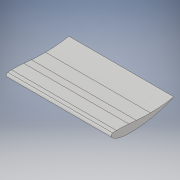
# Autodesk Inventor part: naca97
Saved by Autodesk Inventor 2018.2 (Build 222227000, 227)
## iProperties
Created: 2018-02-23
Part Number: naca97
Material: 一般
Document SubType Name: Modeling
Designer: ku_sk
Density: 1 g/cm^3
Appearance: 既定
Author: ku_sk
Autodesk Inventor part; units mm, degrees
ref_plane "YZ Plane" through (0, 0, 0) normal (1, 0, 0) x (0, 1, 0)
ref_plane "XZ Plane" through (0, 0, 0) normal (0, 1, 0) x (-1, 0, 0)
ref_plane "XY Plane" through (0, 0, 0) normal (0, 0, 1) x (1, 0, 0)
sketch "スケッチ1" plane through (0, 0, 0) normal (0, 1, 0) x (-1, 0, 0)
  arc A0 (-0.3139, 1.7491) -> (-1.4341, -1.0494) centre (0, 0) ccw
  arc A1 (3.0473, 2.0538) -> (-0.3139, 1.7491) centre (3.11, -17.328) ccw
  arc A2 (14.2243, 1.5555) -> (3.0473, 2.0538) centre (3.426, -115.066) ccw
  arc A3 (14.2243, 1.5555) -> (21.0741, 0.9324) centre (210.779, 2124.35) ccw
  arc A4 (21.0741, 0.9324) -> (33.8498, 0.3962) centre (33.144, 136.034) ccw
  arc A5 (33.8498, 0.3962) -> (55, 2.3978) centre (33.229, 119.698) ccw
  arc A6 (-1.4341, -1.0494) -> (-0.1426, -2.3034) centre (2.9, 2.122) ccw
  arc A7 (-0.1426, -2.3034) -> (4.4066, -4.5379) centre (9.743, 12.075) ccw
  arc A8 (4.4066, -4.5379) -> (12.2873, -5.9387) centre (13.508, 23.796) ccw
  arc A9 (12.2873, -5.9387) -> (16.5781, -5.9878) centre (15.261, 66.497) ccw
  arc A10 (16.5781, -5.9878) -> (55, 2.3978) centre (14.7503, 94.6026) ccw
  dimension "d0" = 1.777
  dimension "d2" = 17.328
  dimension "d5" = 115.066
  dimension "d7" = 2124.35
  dimension "d9" = 136.034
  dimension "d10" = 3.11
  dimension "d11" = 3.426
  dimension "d12" = 210.779
  dimension "d13" = 33.144
  dimension "d14" = 33.229
  dimension "d15" = 119.698
  dimension "d16" = 55
  dimension "d17" = 2.9
  dimension "d18" = 2.122
  dimension "d21" = 9.743
  dimension "d22" = 12.075
  dimension "d23" = 13.508
  dimension "d24" = 23.796
  dimension "d25" = 15.261
  dimension "d26" = 66.497
  dimension "d27" = 94.6026
  constraints: 22 point on circle, 11 centre point, 10 tangent, 1 coincident
  measures "d0" radius of A0
  measures "d2" vertical distance of point (0, 0) A1.centre
  measures "d5" vertical distance of point (0, 0) A2.centre
  measures "d7" vertical distance of A3.centre point (0, 0)
  measures "d9" vertical distance of point (0, 0) A4.centre
  measures "d10" horizontal distance of A1.centre point (0, 0)
  measures "d11" horizontal distance of point (0, 0) A2.centre
  measures "d12" horizontal distance of point (0, 0) A3.centre
  measures "d13" horizontal distance of point (0, 0) A4.centre
  measures "d14" horizontal distance of point (0, 0) A5.centre
  measures "d15" vertical distance of point (0, 0) A5.centre
  measures "d16" horizontal distance of A5.end point (0, 0)
  measures "d17" horizontal distance of point (0, 0) A6.centre
  measures "d18" vertical distance of point (0, 0) A6.centre
  measures "d21" horizontal distance of point (0, 0) A7.centre
  measures "d22" vertical distance of point (0, 0) A7.centre
  measures "d23" horizontal distance of point (0, 0) A8.centre
  measures "d24" vertical distance of A8.centre point (0, 0)
  measures "d25" horizontal distance of point (0, 0) A9.centre
  measures "d26" vertical distance of point (0, 0) A9.centre
  measures "d27" vertical distance of point (0, 0) A10.centre
extrude "押し出し1" add sketch "スケッチ1" along normal mid plane 95
